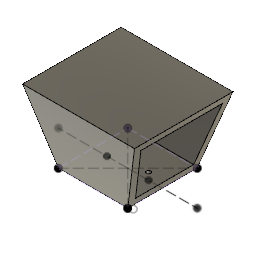
pegboardRester_final (Autodesk Fusion 360 design; units mm, degrees)
Autodesk Fusion 360 part; units mm, degrees
sketch "Sketch1" plane through (0, 0, 0) normal (0, 0, 1) x (1, 0, 0)
  line L0 (0, 0) -> (50, 0)
  line L1 (50, 0) -> (50, 50)
  line L2 (50, 50) -> (0, 50)
  line L3 (0, 50) -> (0, 0)
  line L4 (50, 50) -> (0, 0) construction
  line L5 (0, 50) -> (50, 0) construction
  dimension "d1" = 50
  dimension "d2" = 50
  constraint horizontal L0
  constraint vertical L1
  constraint horizontal L2
  constraint vertical L3
  constraint coincident L0.start L3.end
  measures "d1" distance of L0.start L0.end
  measures "d2" distance of L0.start L2.end
ref_plane "WorkPlane1" through (25, 25, 50) normal (0, 0, 1) x (1, 0, 0)
sketch "Sketch2" plane through (25, 25, 50) normal (0, 0, 1) x (1, 0, 0)
  line L0 (40.2062, -35.3906) -> (-40.512, -35.3906)
  line L1 (-40.512, -35.3906) -> (-40.512, 35.6964)
  line L2 (-40.512, 35.6964) -> (40.2062, 35.6964)
  line L3 (40.2062, 35.6964) -> (40.2062, -35.3906)
  line L4 (40.2062, -35.3906) -> (-40.512, 35.6964) construction
  line L5 (40.2062, 35.6964) -> (-40.512, -35.3906) construction
  constraint horizontal L0
  constraint vertical L1
  constraint horizontal L2
  constraint vertical L3
loft "Loft1" add profiles "Sketch1", "Sketch2" section 1 section 2
shell "Shell2" thickness 5 removed faces 2 at (-10.3413, 33.4353, 33.3333) at (60.1375, 33.4353, 33.3333)
sketch "Sketch3" plane through (0, 0, 0) normal (0, 0, 1) x (1, 0, 0)
  line L0 (0, 0) -> (0, 50) construction
  line L1 (0, 50) -> (50, 50) construction
  line L2 (50, 50) -> (50, 0) construction
  line L3 (50, 0) -> (0, 0) construction
  line L4 (52.5279, 1.4195) -> (50, 0) construction
  line L5 (50, 0) -> (0, 50) construction
  line L6 (0, 0) -> (50, 50) construction
  line L7 (25, 25) -> (-25, 25) construction
  line L8 (25, 25) -> (75, 25) construction
  circle A0 centre (10, 25) radius 1.5
  circle A1 centre (40, 25) radius 1.5
  dimension "d6" = 50
  dimension "d7" = 50
  dimension "d8" = 3
  dimension "d9" = 10
  dimension "d10" = 3
  dimension "d11" = 10
  constraint coincident L2.end L3.start
  constraint coincident L0.end L1.start
  constraint coincident L0.start L3.end
  constraint coincident L1.end L2.start
  constraint midpoint L6 L7.start
  constraint parallel L3 L7
  constraint parallel L7 L8
  constraint coincident L7 A0.centre
  constraint coincident L8 A1.centre
  measures "d6" distance of L7.start L7.end
  measures "d7" distance of L7.start L8.end
  measures "d8" diameter of A0
  measures "d9" distance of L0 A0.centre
  measures "d10" diameter of A1
  measures "d11" distance of L2 A1.centre
extrude "Extrude1" add sketch "Sketch3" against normal blind 5 contours A0
extrude "Extrude2" add sketch "Sketch3" against normal blind 5 contours A1
extrude "Extrude3" cut 1 faces at (40.3665, 25.3401, -5) along direction (0, 0, 1) blind 5
extrude "Extrude4" cut sketch "Sketch3" along normal blind 5 contours A1
extrude "Extrude5" cut 1 faces at (10.4505, 24.7831, -5) along direction (0, 0, 1) blind 10
shell "Shell1" [suppressed]
